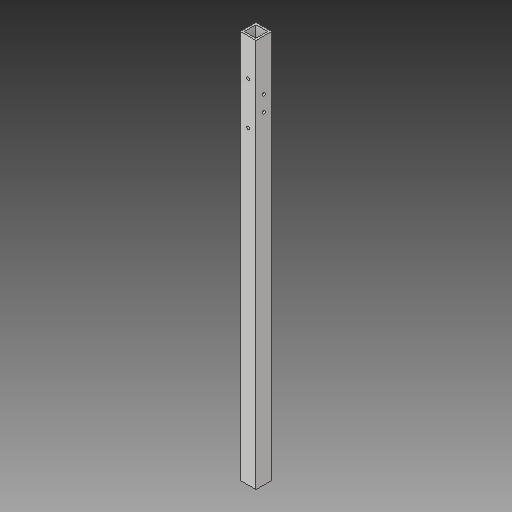
# Autodesk Inventor part: 1x25-topPost
Saved by Autodesk Inventor 2018.2 (Build 222227000, 227)
## iProperties
Created: 2018-02-08
Part Number: 1x25-topPost
Material: Generic
Document SubType Name: Modeling
Designer: steele
Density: 1 g/cm^3
Appearance: Default
Author: steele
Autodesk Inventor part; units mm, degrees
ref_plane "YZ Plane" through (0, 0, 0) normal (1, 0, 0) x (0, 1, 0)
ref_plane "XZ Plane" through (0, 0, 0) normal (0, 1, 0) x (-1, 0, 0)
ref_plane "XY Plane" through (0, 0, 0) normal (0, 0, 1) x (1, 0, 0)
sketch "Sketch1" plane through (0, 0, 0) normal (0, 1, 0) x (-1, 0, 0)
  line L0 (12.7, 12.7) -> (-12.7, 12.7)
  line L1 (-12.7, 12.7) -> (-12.7, -12.7)
  line L2 (-12.7, -12.7) -> (12.7, -12.7)
  line L3 (12.7, -12.7) -> (12.7, 12.7)
  line L4 (12.7, 12.7) -> (-12.7, -12.7) construction
  line L5 (-12.7, 12.7) -> (12.7, -12.7) construction
  line L6 (9.525, 9.525) -> (-9.525, 9.525)
  line L7 (-9.525, 9.525) -> (-9.525, -9.525)
  line L8 (-9.525, -9.525) -> (9.525, -9.525)
  line L9 (9.525, -9.525) -> (9.525, 9.525)
  line L10 (9.525, 9.525) -> (-9.525, -9.525) construction
  line L11 (-9.525, 9.525) -> (9.525, -9.525) construction
  point P0 (0, 0)
  dimension "d0" = 25.4
  dimension "d1" = 3.175
  constraints: 24 end point, 4 midpoint, 4 parallel, 4 perpendicular, 2 horizontal
  measures "d0" distance of L0.start L0.end
  measures "d1" distance between parallel lines of L6 L0
extrude "Extrusion1" add sketch "Sketch1" along normal blind 635
sketch "Sketch2" plane through (12.7, 0, 12.7) normal (1, 0, 0) x (0, 0, -1)
  point P0 (12.7, 552.45)
  point P1 (12.7, 527.05)
hole "Hole1" at (12.7, 552.45, 0) at (12.7, 527.05, 0) direction (-1, 0, 0) diameter 5.1054 depth 3.175
sketch "Sketch3" plane through (-12.7, 0, -12.7) normal (-1, 0, 0) x (0, 0, 1)
  point P0 (12.7, 552.45)
  point P1 (12.7, 527.05)
hole "Hole3" at (-12.7, 552.45, 0) at (-12.7, 527.05, 0) direction (1, 0, 0) diameter 5.1054 depth 3.175
sketch "Sketch6" plane through (12.7, 0, -12.7) normal (0, 0, -1) x (-1, 0, 0)
  point P0 (12.7, 574.675)
hole "Hole8" at (0, 574.675, -12.7) direction (0, 0, 1) diameter 5.08 depth 3.175
sketch "Sketch7" plane through (-12.7, 0, 12.7) normal (0, 0, 1) x (1, 0, 0)
  point P0 (12.7, 574.675)
hole "Hole10" at (0, 574.675, 12.7) direction (0, 0, -1) diameter 5.08 depth 3.175
sketch "Sketch8" plane through (12.7, 0, -12.7) normal (0, 0, -1) x (-1, 0, 0)
  point P0 (12.7, 504.825)
hole "Hole12" at (0, 504.825, -12.7) direction (0, 0, 1) diameter 5.08 depth 3.175
sketch "Sketch9" plane through (-12.7, 0, 12.7) normal (0, 0, 1) x (1, 0, 0)
  point P0 (12.7, 504.825)
hole "Hole14" at (0, 504.825, 12.7) direction (0, 0, -1) diameter 5.08 depth 3.175
body "Solid1"
